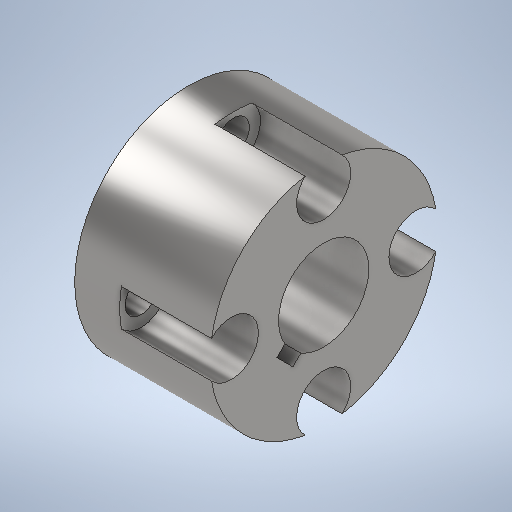
# Autodesk Inventor part: HipCoupler V2
Saved by Autodesk Inventor 2025.1 (Build 291241020, 241B)
## iProperties
Created: 2023-10-20
Part Number: HipCoupler V2
Material: Steel, Mild
Document SubType Name: Modeling
Designer: megan
Density: 7.85 g/cm^3
Appearance: Semi-Polished
Mass: 80.4268 g
Surface Area: 49.7217 cm^2
Volume: 10.2455 cm^3
Author: megan
Autodesk Inventor part; units mm, degrees
ref_plane "YZ Plane" through (0, 0, 0) normal (1, 0, 0) x (0, 1, 0)
sketch "Sketch1" plane through (0, 0, 0) normal (1, 0, 0) x (0, 1, 0)
  circle A0 centre (0, 0) radius 16
  circle A1 centre (0, 13) radius 2
  circle A2 centre (0, -13) radius 2
  circle A3 centre (-13, 0) radius 2
  circle A4 centre (13, 0) radius 2
  circle A5 centre (0, -13) radius 2
  circle A6 centre (0, 13) radius 2
  circle A7 centre (13, 0) radius 2
  circle A8 centre (-13, 0) radius 2
  circle A9 centre (0, 0) radius 6.35
  line L0 (0, -22.4) -> (0, 22.4) projected
  dimension "d0" = 32
  dimension "d1" = 4
  dimension "d2" = 26
  dimension "d3" = 13
  dimension "d6" = 360
  dimension "d8" = 12.7
  constraints: 10 centre point, 2 coincident, 1 equal radius, 17 other
  measures "d0" diameter of A0
  measures "d1" diameter of A1
  measures "d2" distance of A2.centre A1.centre
  measures "d3" distance of point (0, 0) A2.centre
  measures "d8" diameter of A9
extrude "Extrusion1" add sketch "Sketch1" along normal blind 3 contours A0 L0 A2 A9 A1 | L0 A1 A9 A2 A0
sketch "Sketch2" plane through (3, 0, 0) normal (1, 0, 0) x (0, 0, -1)
  circle A0 centre (0, 0) radius 16 projected
  circle A1 centre (13, 0) radius 2 projected
  circle A2 centre (0, 0) radius 6.35 projected
  circle A3 centre (0, -13) radius 2 projected
  circle A4 centre (-13, 0) radius 2 projected
  circle A5 centre (0, 13) radius 2 projected
  circle A6 centre (0, 0) radius 7.5
  dimension "d11" = 15
  constraints: 1 centre point, 1 coincident
  measures "d11" diameter of A6
extrude "Extrusion2" add sketch "Sketch2" along normal blind 10 contours A6
ref_plane "Work Plane1" through (0, 0, 0) normal (0, 0.7071068, -0.7071068) x (-1, 0, 0)
sketch "Sketch6" plane through (3, 0, 0) normal (1, 0, 0) x (0, 0, -1)
  circle A0 centre (0, 0) radius 7.5565
  circle A1 centre (0, 0) radius 6.35 projected
  circle A2 centre (0, 0) radius 7.5 projected
  circle A3 centre (0, 0) radius 6.35 projected
  dimension "d18" = 15.113
  constraints: 1 centre point, 1 coincident
  measures "d18" diameter of A0
sketch "Sketch6 outline for Extrusion4" plane through (3, 0, 0) normal (1, 0, 0) x (0, 0, -1)
  circle A0 centre (0, 0) radius 7.5565
  circle A1 centre (0, 0) radius 7.5
extrude "Extrusion4" add sketch "Sketch6 outline for Extrusion4" along normal up to surface (10 mm away)
sketch "Sketch7" plane through (3, 0, 0) normal (1, 0, 0) x (0, 0, -1)
  circle A0 centre (-13, 0) radius 2
  circle A1 centre (-13, 0) radius 3
  circle A2 centre (0, 13) radius 2
  circle A3 centre (0, 13) radius 3
  circle A4 centre (13, 0) radius 2
  circle A5 centre (13, 0) radius 2.999819
  circle A6 centre (0, -13) radius 2
  circle A7 centre (0, -13) radius 3
  circle A8 centre (0, 0) radius 7.5565
  circle A9 centre (0, 0) radius 16
  circle A10 centre (0, 13) radius 3.81
  circle A11 centre (-13, 0) radius 3.81
  circle A12 centre (0, -13) radius 3.81
  circle A13 centre (13, 0) radius 3.81
  line L0 (-13, 3.81) -> (-15.539752, 3.81)
  line L1 (-13, -3.81) -> (-15.539752, -3.81)
  line L2 (-3.81, -13) -> (-3.81, -15.539752)
  line L3 (3.81, -13) -> (3.81, -15.539752)
  line L4 (13, -3.81) -> (15.539752, -3.81)
  line L5 (13, 3.81) -> (15.539752, 3.81)
  line L6 (-3.81, 13) -> (-3.81, 15.539752)
  line L7 (3.81, 13) -> (3.81, 15.539752)
  point P0 (15.787842, -2.596928)
  point P1 (15.787842, 2.596928)
  point P2 (2.596928, 15.787842)
  point P3 (-2.596928, 15.787842)
  point P4 (-15.787842, 2.596928)
  point P5 (-15.787842, -2.596928)
  point P6 (-2.596928, -15.787842)
  point P7 (2.596928, -15.787842)
  dimension "d21" = 7.62
  dimension "d22" = 7.62
  dimension "d23" = 7.62
  dimension "d24" = 7.62
  constraints: 16 end point, 8 centre point, 8 coincident, 8 point on circle, 6 point on line, 2 parallel, 1 horizontal, 1 perpendicular, 9 other
  measures "d21" diameter of A10
  measures "d22" diameter of A11
  measures "d23" diameter of A12
  measures "d24" diameter of A13
extrude "Extrusion5" add sketch "Sketch7" along normal up to surface (10 mm away) contours A1 | A9 A11 | A9 L0 A11 | A11 L1 A9 | A9 L6 A10 L7 L5 A13 L4 L3 A12 L2 L1 A11 L0 | A9 A10 L6 | L2 A12 A9 | A3 | A9 A10 | A7 | A12 A9 | A9 L7 A10 | A12 L3 A9 | A9 A13 L5 | L4 A13 A9 | A5 | A9 A13 picked at (-9.491842, -0.282602) picked at (3.503096, 12.696069) picked at (3.503096, -12.696069) picked at (12.57554, -3.495745)
sketch "Sketch8" plane through (13, 0, 0) normal (1, 0, 0) x (0, 0, -1)
  circle A0 centre (0, -13) radius 2
  circle A1 centre (-13, 0) radius 2
  line L0 (-4.495748, -4.495171) -> (-3.429275, -5.671093)
  line L1 (-4.495748, -4.495171) -> (-5.56222, -3.319249)
  circle A2 centre (0, 0) radius 6.35
  line L2 (-5.56222, -3.319249) -> (-5.465977, -3.231964)
  line L3 (-3.429275, -5.671093) -> (-3.214472, -5.476283)
  line L4 (-3.214472, -5.476283) -> (-5.45172, -3.219033)
  line L5 (-5.45172, -3.219033) -> (-6.579236, -4.336559)
  line L6 (-3.214472, -5.476283) -> (-4.341988, -6.593808)
  line L7 (-6.579236, -4.336559) -> (-4.344185, -6.591592)
  line L8 (-4.341988, -6.593808) -> (-4.344185, -6.591592)
  dimension "d27" = 1.5875
  dimension "d28" = 1.5875
  dimension "d29" = 1.5875
  dimension "d30" = 1.5875
  dimension "d31" = 90
  dimension "d32" = 0
  dimension "d33" = 90
  dimension "d34" = 3.175
  dimension "d35" = 90
  constraints: 18 end point, 2 point on circle, 1 perpendicular
  measures "d27" distance of L0.start L0.end
  measures "d28" distance of L0.start L1.end
  measures "d29" distance of L4.end L5.end
  measures "d30" distance of L3.end L6.end
  measures "d31" angle of L5 L7
  measures "d32" distance edge to line of A2 L1
  measures "d33" angle of L5 L4
  measures "d34" distance of L5.end L7.end
  measures "d35" angle of L4 L6
extrude "Extrusion6" cut sketch "Sketch8" against normal up to surface (13 mm away) contours L1 A2 L3 L0 | L0 L3 L6 L8 L7 L5 L1 | L1 L5 A2 | A2 L5 L4 picked at (-4.633855, -4.096279)
sketch "Sketch9" plane through (13, 0, 0) normal (1, 0, 0) x (0, 0, -1)
  line L0 (-3.214472, -5.476283) -> (-4.341988, -6.593808)
  line L1 (-4.341988, -6.593808) -> (-6.579236, -4.336559)
  line L2 (-6.579236, -4.336559) -> (-5.46553, -3.232721)
  arc A0 (-3.214472, -5.476283) -> (-5.46553, -3.232721) centre (0, 0) ccw
  circle A1 centre (0, 13) radius 2
  circle A2 centre (-13, 0) radius 2
  circle A3 centre (0, -13) radius 2
  circle A4 centre (13, 0) radius 2
  circle A5 centre (0, 0) radius 16
extrude "Extrusion7" add sketch "Sketch9" along normal blind 6.0452
sketch "Sketch10" plane through (19.0452, 0, 0) normal (1, 0, 0) x (0, 0, -1)
  circle A0 centre (13, 0) radius 2 projected
  point P0 (0, 0)
  constraints: 1 coincident
hole "Hole1" at (19.0452, 0, -13) direction (-1, 0, 0) diameter 4.4958 end through all counterbore diameter 7.62 counterbore depth 12.7 clearance for "Hex Machine Screw" size "#8" standard "Ansi Unified Screw Threads"
sketch "Sketch11" plane through (19.0452, 0, 0) normal (1, 0, 0) x (0, 0, -1)
  circle A0 centre (0, 13) radius 2 projected
  point P0 (0, 0)
  point P1 (0, 13)
  constraints: 1 coincident
hole "Hole2" at (19.0452, 13, 0) direction (-1, 0, 0) diameter 4.4958 end through all counterbore diameter 7.62 counterbore depth 12.7 clearance for "Hex Machine Screw" size "#8" standard "Ansi Unified Screw Threads"
sketch "Sketch12" plane through (19.0452, 0, 0) normal (1, 0, 0) x (0, 0, -1)
  circle A0 centre (-13, 0) radius 2 projected
  point P0 (0, 0)
  constraints: 1 coincident
hole "Hole3" at (19.0452, 0, 13) direction (-1, 0, 0) diameter 4.4958 end through all counterbore diameter 7.62 counterbore depth 12.7 clearance for "Hex Machine Screw" size "#8" standard "Ansi Unified Screw Threads"
sketch "Sketch13" plane through (19.0452, 0, 0) normal (1, 0, 0) x (0, 0, -1)
  circle A0 centre (0, -13) radius 2 projected
  point P0 (0, 0)
  point P1 (0, -13)
  constraints: 1 coincident
hole "Hole4" at (19.0452, -13, 0) direction (-1, 0, 0) diameter 4.4958 end through all counterbore diameter 7.62 counterbore depth 12.7 clearance for "Hex Machine Screw" size "#8" standard "Ansi Unified Screw Threads"
body "Solid1"
